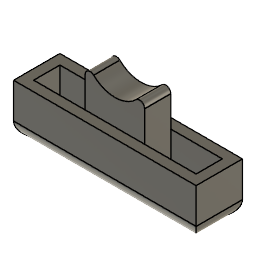
Cap 3 (Autodesk Fusion 360 design; units mm, degrees)
Autodesk Fusion 360 part; units mm, degrees
sketch "Sketch1" plane through (0, 0, 0) normal (0, 0, 1) x (1, 0, 0)
  line L0 (0, 0) -> (32.2, 0)
  line L1 (32.2, 0) -> (32.2, 5.2)
  line L2 (32.2, 5.2) -> (0, 5.2)
  line L3 (0, 5.2) -> (0, 0)
  line L4 (-2, -2) -> (34.2, -2)
  line L5 (34.2, -2) -> (34.2, 7.2)
  line L6 (34.2, 7.2) -> (-2, 7.2)
  line L7 (-2, 7.2) -> (-2, -2)
  line L8 (10.2, 5.2) -> (22, 5.2)
  line L9 (22, 5.2) -> (22, 0)
  line L10 (22, 0) -> (10.2, 0)
  line L11 (10.2, 0) -> (10.2, 5.2)
  dimension "d1" = 5.2
  dimension "d2" = 32.2
  dimension "d3" = 2
  dimension "d4" = 10.2
  dimension "d5" = 10.2
  constraint horizontal L0
  constraint vertical L1
  constraint horizontal L2
  constraint vertical L3
  constraint coincident L0.start L3.end
  constraint horizontal L8
  constraint vertical L9
  constraint horizontal L10
  constraint vertical L11
  constraint coincident L0 L9.end
  constraint coincident L2 L8.start
  measures "d1" distance of L0 L2
  measures "d2" distance of L1 L3
  measures "d4" distance of L3 L11
  measures "d5" distance of L1 L9
extrude "Extrude1" add sketch "Sketch1" along normal blind 8
extrude "Extrude2" add sketch "Sketch1" against normal blind 2 contours L0 L2 L3 L11 | L0 L2 L8 L9 L10 L11 | L0 L1 L2 L9 | L4 L5 L6 L7
extrude "Extrude3" add sketch "Sketch1" along normal blind 18 contours L0 L2 L8 L9 L10 L11
sketch "Sketch2" plane through (0, 5.2, 0) normal (0, 1, 0) x (-1, 0, 0)
  line L0 (-22, 8) -> (-10.2, 8)
  line L1 (-10.2, 8) -> (-10.2, 18)
  line L2 (-10.2, 18) -> (-22, 18)
  line L3 (-22, 18) -> (-22, 8)
  arc A0 (-22, 18) -> (-10.2, 18) centre (-16.1, 19.0909) ccw
  dimension "d19" = 6
  constraint coincident L2.end L3.start
  constraint coincident L1.end L2.start
  measures "d19" radius of A0
extrude "Extrude4" cut sketch "Sketch2" against normal up to surface (5.2 mm away) contours L2 A0
fillet "Fillet1" radius 3 4 edges at (-2, 2.6, -2) (16.1, 7.2, -2) (34.2, 2.6, -2) (16.1, -2, -2)
fillet "Fillet3" radius 1 2 edges at (10.2, 2.6, 18) (22, 2.6, 18)
